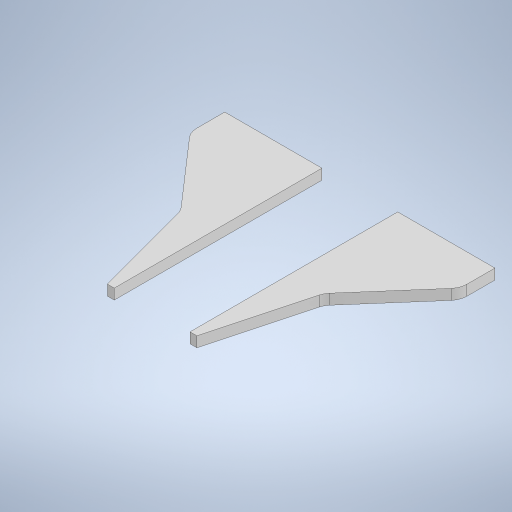
# Autodesk Inventor part: wings
Saved by Autodesk Inventor 2024 (Build 280153000, 153)
## iProperties
Created: 2023-06-07
Part Number: wings
Material: Generic
Document SubType Name: Modeling
Designer: tamiz
Density: 1 g/cm^3
Appearance: Default
Author: tamiz
Autodesk Inventor part; units mm, degrees
ref_plane "YZ Plane" through (0, 0, 0) normal (1, 0, 0) x (0, 1, 0)
ref_plane "XZ Plane" through (0, 0, 0) normal (0, 1, 0) x (-1, 0, 0)
ref_plane "XY Plane" through (0, 0, 0) normal (0, 0, 1) x (1, 0, 0)
ref_plane "Work Plane8" through (-3200.4, -2400.3, 0) normal (0, -1, 0) x (1, 0, 0)
sketch "Sketch14" plane through (-3200.4, -2400.3, 0) normal (0, -1, 0) x (1, 0, 0)
  line L0 (-744.5402, 0) -> (-3019.8458, -8491.5564)
  line L1 (-744.5402, 0) -> (8046.5659, 0) construction
  line L2 (-8695.944, -18288) -> (-8695.944, -15810.9375)
  line L3 (-8320.8116, -14809.5987) -> (-3343.0492, -9098.4549)
  arc A0 (-3343.0492, -9098.4549) -> (-3019.8458, -8491.5564) centre (-4491.9168, -8097.1161) ccw
  arc A1 (-8320.8116, -14809.5987) -> (-8695.944, -15810.9375) centre (-7171.944, -15810.9375) ccw
  line L4 (7145.3402, 0) -> (9420.6458, -8491.5564)
  line L5 (15096.744, -18288) -> (15096.744, -15810.9375)
  line L6 (14721.6116, -14809.5987) -> (9743.8492, -9098.4549)
  arc A2 (15096.744, -15810.9375) -> (14721.6116, -14809.5987) centre (13572.744, -15810.9375) ccw
  arc A3 (9420.6458, -8491.5564) -> (9743.8492, -9098.4549) centre (10892.7168, -8097.1161) ccw
  line L7 (-8695.944, -18288) -> (-134.9402, -18288)
  line L8 (15096.744, -18288) -> (6535.7402, -18288)
  line L9 (-744.5402, 0) -> (-134.9402, 0)
  line L10 (-134.9402, 0) -> (-134.9402, -18288)
  line L11 (7145.3402, 0) -> (6535.7402, 0)
  line L12 (6535.7402, 0) -> (6535.7402, -18288)
  point P0 (3200.4, -18288)
  point P1 (-3111.1815, -8832.4258)
  point P2 (-8695.944, -15240)
  dimension "d47" = 9144
  dimension "d48" = 105
  dimension "d49" = 3048
  dimension "d50" = 1524
  dimension "d51" = 1524
  dimension "d60" = 609.6
  dimension "d61" = 609.6
  constraints: 26 end point, 8 point on circle, 6 point on line, 4 centre point, 4 tangent, 2 perpendicular, 1 equal length, 1 horizontal, 1 vertical
  measures "d47" distance of L0.start point (-3111.182, -8832.426)
  measures "d48" angle of L0 L1
  measures "d49" distance of L2.start point (-8695.944, -15240)
  measures "d50" radius of A0
  measures "d51" radius of A1
  measures "d60" distance of L0.start L9.end
  measures "d61" distance of L4.start L11.end
extrude "Extrusion9" add sketch "Sketch14" along normal blind 914.4
body "Solid1"
